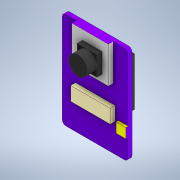
# Autodesk Inventor part: esp32-cam-sp
Saved by Autodesk Inventor 2020 (Build 240168000, 168)
## iProperties
Created: 2020-11-03
Part Number: esp32-cam-sp
Material: Generic
Document SubType Name: Modeling
Designer: alnwlsn
Density: 1 g/cm^3
Appearance: Default
Author: alnwlsn
Autodesk Inventor part; units mm, degrees
ref_plane "YZ Plane" through (0, 0, 0) normal (1, 0, 0) x (0, 1, 0)
ref_plane "XZ Plane" through (0, 0, 0) normal (0, 1, 0) x (-1, 0, 0)
ref_plane "XY Plane" through (0, 0, 0) normal (0, 0, 1) x (1, 0, 0)
sketch "Sketch1" plane through (0, 0, 0) normal (0, 0, 1) x (1, 0, 0)
  line L0 (1.5, 0) -> (25.67, 0)
  line L1 (27.17, 1.5) -> (27.17, 38.5)
  line L2 (25.67, 40) -> (1.5, 40)
  line L3 (0, 38.5) -> (0, 1.5)
  arc A0 (1.5, 40) -> (0, 38.5) centre (1.5, 38.5) ccw
  arc A1 (27.17, 38.5) -> (25.67, 40) centre (25.67, 38.5) ccw
  arc A2 (25.67, 0) -> (27.17, 1.5) centre (25.67, 1.5) ccw
  arc A3 (0, 1.5) -> (1.5, 0) centre (1.5, 1.5) ccw
  point P0 (0, 0)
  point P1 (27.17, 40)
  point P2 (0, 40)
  dimension "d0" = 40
  dimension "d1" = 27.17
  dimension "d2" = 1.5
  constraints: 8 end point, 8 point on circle, 8 tangent, 6 point on line, 4 centre point, 3 equal radius, 2 parallel, 1 horizontal, 1 perpendicular
  measures "d0" distance of point (0, 40) point (0, 0)
  measures "d1" distance of point (27.17, 40) point (0, 40)
  measures "d2" radius of A0
extrude "Extrusion1" add sketch "Sketch1" along normal blind 1.6
sketch "Sketch2" plane through (0, 0, 1.6) normal (0, 0, 1) x (1, 0, 0)
  line L0 (25.67, 40) -> (1.5, 40) projected
  line L1 (6, 40) -> (21, 40)
  line L2 (21, 40) -> (21, 25)
  line L3 (21, 25) -> (6, 25)
  line L4 (6, 25) -> (6, 40)
  line L5 (0, 38.5) -> (0, 1.5) projected
  line L6 (5.5, 17.5) -> (21.8, 17.5)
  line L7 (21.8, 17.5) -> (21.8, 11.8)
  line L8 (21.8, 11.8) -> (5.5, 11.8)
  line L9 (5.5, 11.8) -> (5.5, 17.5)
  line L10 (1.5, 0) -> (25.67, 0) projected
  line L11 (27.17, 1.5) -> (27.17, 38.5) projected
  line L12 (27.17, 12.8) -> (23.17, 12.8)
  line L13 (23.17, 12.8) -> (23.17, 8.8)
  line L14 (23.17, 8.8) -> (27.17, 8.8)
  line L15 (27.17, 8.8) -> (27.17, 12.8)
  point P0 (0, 0)
  dimension "d5" = 15
  dimension "d6" = 15
  dimension "d7" = 6
  dimension "d8" = 5.7
  dimension "d9" = 16.3
  dimension "d10" = 5.5
  dimension "d11" = 11.8
  dimension "d12" = 4
  dimension "d13" = 4
  dimension "d14" = 8.8
  constraints: 24 end point, 6 parallel, 3 horizontal, 3 perpendicular, 2 point on line
  measures "d5" distance of L2.end L3.end
  measures "d6" distance of L3.end L1.start
  measures "d7" distance between parallel lines of L5 L4
  measures "d8" distance between parallel lines of L8 L6
  measures "d9" distance of L7.end L8.end
  measures "d10" distance between parallel lines of L5 L9
  measures "d11" distance between parallel lines of L10 L8
  measures "d12" distance between parallel lines of L14 L12
  measures "d13" distance of L12.start L12.end
  measures "d14" distance between parallel lines of L10 L14
extrude "Extrusion2" add sketch "Sketch2" along normal blind 2 contours L2 L3 L4 L0
extrude "Extrusion3" add sketch "Sketch2" along normal blind 2 contours L6 L7 L8 L9
extrude "Extrusion4" add sketch "Sketch2" along normal blind 1 contours L14 L13 L12 L11
sketch "Sketch3" plane through (0, 0, 3.6) normal (0, 0, 1) x (1, 0, 0)
  line L0 (10.37, 36.1) -> (18.47, 36.1)
  line L1 (18.47, 36.1) -> (18.47, 28)
  line L2 (18.47, 28) -> (10.37, 28)
  line L3 (10.37, 28) -> (10.37, 36.1)
  line L4 (25.67, 40) -> (21, 40) projected
  line L5 (27.17, 12.8) -> (27.17, 38.5) projected
  point P0 (0, 0)
  dimension "d21" = 8.1
  dimension "d22" = 8.1
  dimension "d23" = 3.9
  dimension "d24" = 8.7
  constraints: 8 end point, 2 parallel, 1 horizontal, 1 perpendicular
  measures "d21" distance of L2.end L0.start
  measures "d22" distance of L0.start L0.end
  measures "d23" distance between parallel lines of L4 L0
  measures "d24" distance between parallel lines of L5 L1
extrude "Extrusion5" add sketch "Sketch3" along normal blind 2.2
sketch "Sketch4" plane through (0, 0, 5.8) normal (0, 0, 1) x (1, 0, 0)
  circle A0 centre (14.42, 32.05) radius 3.9
  circle A1 centre (14.42, 32.05) radius 4.05
  line L0 (18.47, 36.1) -> (10.37, 36.1) projected
  line L1 (18.47, 28) -> (18.47, 36.1) projected
  point P0 (0, 0)
  dimension "d27" = 7.8
  constraints: 2 centre point, 2 tangent, 1 coincident
  measures "d27" diameter of A0
extrude "Extrusion6" add sketch "Sketch4" along normal blind 3.7 contours A0
sketch "Sketch5" plane through (0, 0, 0) normal (0, 0, -1) x (-1, 0, 0)
  line L0 (-1.035, 16.4) -> (-3.035, 16.4)
  line L1 (-3.035, 16.4) -> (-3.035, 36.4)
  line L2 (-3.035, 36.4) -> (-1.035, 36.4)
  line L3 (-1.035, 36.4) -> (-1.035, 16.4)
  line L4 (-24.135, 16.4) -> (-26.135, 16.4)
  line L5 (-26.135, 16.4) -> (-26.135, 36.4)
  line L6 (-26.135, 36.4) -> (-24.135, 36.4)
  line L7 (-24.135, 36.4) -> (-24.135, 16.4)
  line L8 (0, 38.5) -> (0, 1.5) projected
  line L9 (-27.17, 1.5) -> (-27.17, 38.5) projected
  line L10 (-1.5, 0) -> (-25.67, 0) projected
  line L11 (-25.67, 40) -> (-1.5, 40) projected
  point P0 (0, 0)
  dimension "d30" = 25.1
  dimension "d31" = 2
  dimension "d32" = 1.035
  dimension "d33" = 1.035
  dimension "d36" = 3.6
  dimension "d39" = 20
  constraints: 16 end point, 4 parallel, 2 horizontal, 2 perpendicular, 2 point on line, 1 collinear
  measures "d30" distance between parallel lines of L5 L3
  measures "d31" distance of L0.start L0.end
  measures "d32" distance between parallel lines of L8 L3
  measures "d33" distance between parallel lines of L9 L5
  measures "d36" distance between parallel lines of L11 L2
  measures "d39" distance of L6.end L4.start
extrude "Extrusion7" add sketch "Sketch5" along normal blind 2
body "Solid1"
